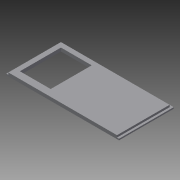
# Autodesk Inventor part: Receiver Case top
Saved by Autodesk Inventor 2014 SP1 (Build 180222100, 222)
## iProperties
Created: 2014-05-12
Part Number: Receiver Case top
Material: Generic
Document SubType Name: Modeling
Designer: Alex
Density: 1 g/cm^3
Appearance: Default
Author: Alex
Autodesk Inventor part; units mm, degrees
ref_plane "YZ Plane" through (0, 0, 0) normal (1, 0, 0) x (0, 1, 0)
ref_plane "XZ Plane" through (0, 0, 0) normal (0, 1, 0) x (-1, 0, 0)
ref_plane "XY Plane" through (0, 0, 0) normal (0, 0, 1) x (1, 0, 0)
sketch "Sketch1" plane through (0, 0, 0) normal (0, 0, 1) x (1, 0, 0)
  line L0 (0, 0) -> (140, 0)
  line L1 (140, 0) -> (140, 80)
  line L2 (140, 80) -> (0, 80)
  line L3 (0, 80) -> (0, 0)
  dimension "d0" = 140
  dimension "d1" = 80
  constraints: 8 end point, 2 parallel, 1 horizontal, 1 perpendicular
  measures "d0" distance of L2.end L1.end
  measures "d1" distance of L1.end L0.end
extrude "Extrusion1" add sketch "Sketch1" along normal blind 2
sketch "Sketch2" plane through (0, 0, 2) normal (0, 0, 1) x (1, 0, 0)
  line L0 (0, 80) -> (2, 80)
  line L1 (2, 80) -> (2, 78)
  line L2 (2, 78) -> (0, 78)
  line L3 (0, 78) -> (0, 80)
  line L4 (2, 78) -> (138, 78)
  line L5 (138, 78) -> (138, 2)
  line L6 (138, 2) -> (2, 2)
  line L7 (2, 2) -> (2, 78)
  dimension "d4" = 2
  dimension "d5" = 2
  dimension "d6" = 136
  dimension "d7" = 76
  constraints: 16 end point, 4 parallel, 2 horizontal, 2 perpendicular
  measures "d4" distance of L1.end L2.end
  measures "d5" distance of L0.end L1.end
  measures "d6" distance of L5.end L6.end
  measures "d7" distance of L4.end L5.end
extrude "Extrusion2" add sketch "Sketch2" along normal blind 3 contours L4 L5 L6 L7
sketch "Sketch3" plane through (0, 0, 2) normal (0, 0, 1) x (1, 0, 0)
  line L0 (0, 0) -> (140, 0) projected
  line L1 (2, 2) -> (138, 2)
  line L2 (138, 2) -> (138, 0)
  line L3 (138, 0) -> (2, 0)
  line L4 (2, 0) -> (2, 2)
  constraints: 8 end point, 2 parallel, 1 horizontal, 1 perpendicular, 1 point on line
extrude "Extrusion3" add sketch "Sketch3" along normal blind 3
sketch "Sketch4" plane through (0, 0, 0) normal (0, 0, -1) x (-1, 0, 0)
  line L0 (0, 0) -> (-140, 0) projected
  line L1 (0, 80) -> (0, 0) projected
  line L2 (-140, 0) -> (0, 0)
  line L3 (0, 0) -> (0, 1)
  line L4 (0, 1) -> (-140, 1)
  line L5 (-140, 1) -> (-140, 0)
  dimension "d12" = 1
  constraints: 8 end point, 2 parallel, 1 horizontal, 1 perpendicular, 1 point on line
  measures "d12" distance of L3.end L2.end
extrude "Extrusion4" cut sketch "Sketch4" against normal blind 7.5
sketch "Sketch5" plane through (0, 0, 0) normal (0, 0, -1) x (-1, 0, 0)
  line L0 (-140, 80) -> (0, 80)
  line L1 (0, 80) -> (0, 81)
  line L2 (0, 81) -> (-140, 81)
  line L3 (-140, 81) -> (-140, 80)
  point P0 (0, 0)
  dimension "d15" = 1
  constraints: 8 end point, 2 parallel, 1 horizontal, 1 perpendicular
  measures "d15" distance of L1.end L0.end
extrude "Extrusion5" add sketch "Sketch5" against normal blind 2
sketch "Sketch6" plane through (0, 0, 5) normal (0, 0, 1) x (1, 0, 0)
  line L0 (138, 78) -> (2, 78) projected
  line L1 (2, 1) -> (3, 1)
  line L2 (3, 1) -> (3, 78)
  line L3 (3, 78) -> (2, 78)
  line L4 (2, 78) -> (2, 1)
  line L5 (138, 1) -> (137, 1)
  line L6 (137, 1) -> (137, 78)
  line L7 (137, 78) -> (138, 78)
  line L8 (138, 78) -> (138, 1)
  point P0 (0, 0)
  dimension "d18" = 1
  dimension "d19" = 1
  constraints: 16 end point, 4 parallel, 2 horizontal, 2 perpendicular, 2 point on line
  measures "d18" distance of L3.end L2.end
  measures "d19" distance of L6.end L7.end
extrude "Extrusion6" cut sketch "Sketch6" against normal blind 3
sketch "Sketch7" plane through (0, 0, 0) normal (0, 0, -1) x (-1, 0, 0)
  line L0 (-140, 1) -> (0, 1) projected
  line L1 (0, 1) -> (0, 81) projected
  line L2 (0, 81) -> (-140, 81) projected
  line L3 (-140, 1) -> (-140, 81) projected
  line L4 (0, 1) -> (-165, 1)
  line L5 (-165, 1) -> (-165, 81)
  line L6 (-165, 81) -> (0, 81)
  line L7 (0, 81) -> (0, 1)
  point P0 (0, 0)
  dimension "d22" = 165
  constraints: 8 end point, 2 parallel, 1 horizontal, 1 perpendicular
  measures "d22" distance of L5.end L6.end
extrude "Extrusion7" add sketch "Sketch7" against normal blind 2 contours L4 L5 L6 L3
sketch "Sketch9" plane through (0, 0, 2) normal (0, 0, 1) x (1, 0, 0)
  line L0 (137, 1) -> (162, 1)
  line L1 (162, 1) -> (162, 78)
  line L2 (162, 78) -> (137, 78)
  line L3 (137, 78) -> (137, 1)
  point P0 (0, 0)
  dimension "d25" = 25
  constraints: 8 end point, 2 parallel, 1 horizontal, 1 perpendicular
  measures "d25" distance of L2.end L1.end
extrude "Extrusion8" add sketch "Sketch9" along normal blind 3
sketch "Sketch10" plane through (0, 0, 0) normal (0, 0, -1) x (-1, 0, 0)
  line L0 (0, 1) -> (-10, 1)
  line L1 (-10, 1) -> (-10, 11)
  line L2 (-10, 11) -> (0, 11)
  line L3 (0, 11) -> (0, 1)
  line L4 (0, 81) -> (-10, 81)
  line L5 (-10, 81) -> (-10, 71)
  line L6 (-10, 71) -> (0, 71)
  line L7 (0, 71) -> (0, 81)
  line L8 (-10, 71) -> (-55, 71)
  line L9 (-55, 71) -> (-55, 11)
  line L10 (-55, 11) -> (-10, 11)
  line L11 (-10, 11) -> (-10, 71)
  point P0 (0, 0)
  dimension "d28" = 10
  dimension "d29" = 10
  dimension "d30" = 10
  dimension "d31" = 10
  dimension "d32" = 45
  constraints: 24 end point, 6 parallel, 3 horizontal, 3 perpendicular
  measures "d28" distance of L1.end L2.end
  measures "d29" distance of L0.end L1.end
  measures "d30" distance of L6.end L5.end
  measures "d31" distance of L5.end L4.end
  measures "d32" distance of L10.end L9.end
extrude "Extrusion9" cut sketch "Sketch10" against normal blind 10.25 contours L10 L9 L8 L11
body "Solid1"
